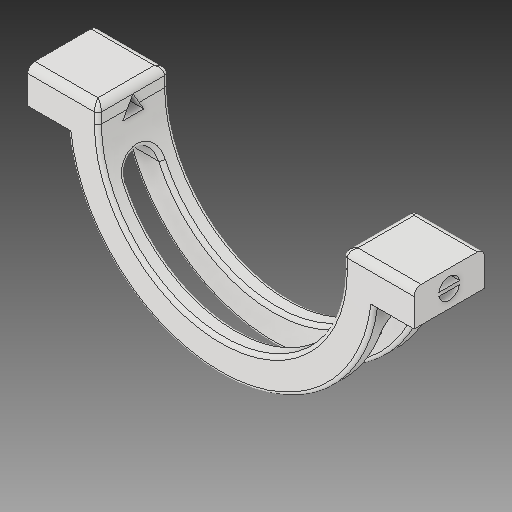
# Autodesk Inventor part: TopCircleArm
Saved by Autodesk Inventor 2017 (Build 210142000, 142)
## iProperties
Created: 2017-02-18
Part Number: TopCircleArm
Material: ABS Plastic
Document SubType Name: Modeling
Designer: aribu
Density: 1.06 g/cm^3
Appearance: Smooth - White
Mass: 19.458 g
Surface Area: 97.5745 cm^2
Volume: 18.3566 cm^3
Author: aribu
Autodesk Inventor part; units mm, degrees
ref_plane "YZ Plane" through (0, 0, 0) normal (1, 0, 0) x (0, 1, 0)
ref_plane "XZ Plane" through (0, 0, 0) normal (0, 1, 0) x (-1, 0, 0)
ref_plane "XY Plane" through (0, 0, 0) normal (0, 0, 1) x (1, 0, 0)
sketch "Sketch1" plane through (0, 0, 0) normal (0, 0, 1) x (1, 0, 0)
  arc A0 (-35, 0) -> (35, 0) centre (0, 0) ccw
  arc A1 (-43.715, -5) -> (43.715, -5) centre (0, 0) ccw
  line L0 (-35, 0) -> (-35, 5)
  line L1 (35, 0) -> (35, 5)
  line L2 (-35, 5) -> (-55, 5)
  line L3 (-55, 5) -> (-55, -5)
  line L4 (-55, -5) -> (-43.715, -5)
  line L5 (35, 5) -> (55, 5)
  line L6 (55, 5) -> (55, -5)
  line L7 (55, -5) -> (43.715, -5)
  dimension "d0" = 70
  dimension "d1" = 88
  dimension "d12" = 20
  dimension "d13" = 20
  dimension "d27" = 10
  dimension "d28" = 10
  constraints: 16 end point, 4 perpendicular, 4 point on circle, 2 centre point, 2 coincident, 2 tangent, 1 horizontal, 1 vertical
  measures "d0" diameter of A0
  measures "d1" diameter of A1
  measures "d12" distance of L0.end L2.end
  measures "d13" distance of L1.end L5.end
  measures "d27" distance of L5.end L6.end
  measures "d28" distance of L2.end L3.end
extrude "Extrusion1" add sketch "Sketch1" along normal blind 20
sketch "Sketch2" plane through (55, -5, 0) normal (1, 0, 0) x (0, 0, -1)
  arc A0 (-5, -10) -> (-15, -10) centre (-10, -10) ccw
  line L0 (0, 10) -> (0, 0)
  line L1 (0, 0) -> (-10, 0)
  line L2 (-15, -10) -> (-15, -42.0097)
  line L3 (-15, -42.0097) -> (-5, -42.0097)
  line L4 (-5, -42.0097) -> (-5, -10)
  line L5 (0, 0) -> (-20, 0) projected
  line L6 (0, 10) -> (0, 0) projected
  dimension "d6" = 10
  dimension "d7" = 10
  dimension "d8" = 10
  dimension "d14" = 0
  dimension "d15" = 0
  dimension "d16" = 10
  constraints: 10 end point, 2 point on circle, 2 tangent, 1 centre point, 1 perpendicular, 1 vertical
  measures "d6" diameter of A0
  measures "d7" distance from line of L0 A0.centre
  measures "d8" distance from line of L1 A0.centre
  measures "d14" distance between parallel lines of L1 L5
  measures "d15" distance between parallel lines of L6 L0
  measures "d16" distance of L2.end L3.end
extrude "Extrusion2" cut sketch "Sketch2" against normal blind 120
fillet "Fillet1" radius 1 16 edges at (33.541, -10, 9.9987) (0, -35, 15) (-33.541, -10, 9.9987) (0, -35, 5) (-42.8486, -10, 9.9954) (0, -44, 15) (42.8486, -10, 9.9954) (0, -44, 5) (0, -44, 20) (0, -44, 0) (35, 2.5, 0) (-35, 2.5, 0) (0, -35, 0) (-35, 2.5, 20) (35, 2.5, 20) (0, -35, 20)
sketch "Sketch3" plane through (55, -5, 0) normal (1, 0, 0) x (0, 0, -1)
  line L0 (-20, 0) -> (-20, 10) projected
  line L1 (0, 10) -> (-20, 10) projected
  line L2 (-12.9139, 4.5) -> (-7.0861, 4.5)
  line L3 (-7.052, 5.5) -> (-12.948, 5.5)
  arc A0 (-12.9139, 4.5) -> (-7.0861, 4.5) centre (-10, 5) ccw
  arc A1 (-7.052, 5.5) -> (-12.948, 5.5) centre (-10, 5) ccw
  point P0 (0, 5)
  dimension "d18" = 10
  dimension "d19" = 5
  dimension "d35" = 1
  dimension "d36" = 0.5
  constraints: 4 end point, 4 point on circle, 2 centre point, 1 horizontal, 1 parallel
  measures "d18" distance from line of L0 A0.centre
  measures "d19" distance from line of A0.centre L1
  measures "d35" distance between parallel lines of L3 L2
  measures "d36" distance from line of L3 A0.centre
extrude "Extrusion3" cut sketch "Sketch3" against normal blind 25
fillet "Fillet2" radius 2 10 edges at (-35.2929, 5, 0.2929) (-35, 5, 10) (-35.2929, 5, 19.7071) (-45.5, 5, 20) (-45.5, 5, 0) (35.2929, 5, 0.2929) (35, 5, 10) (35.2929, 5, 19.7071) (45.5, 5, 20) (45.5, 5, 0)
sketch "Sketch4" plane through (-55, -5, 0) normal (-1, 0, 0) x (0, 0, 1)
  line L0 (19, 8) -> (1, 8) projected
  line L1 (10, 8) -> (7, 2.8038)
  line L2 (7, 2.8038) -> (13, 2.8038)
  line L3 (13, 2.8038) -> (10, 8)
  point P0 (0, 5)
  dimension "d30" = 6
  dimension "d31" = 6
  dimension "d32" = 6
  constraints: 6 end point, 1 horizontal, 1 midpoint
  measures "d30" distance of L2.end L1.start
  measures "d31" distance of L1.start L1.end
  measures "d32" distance of L1.end L2.end
extrude "Extrusion4" cut sketch "Sketch4" against normal blind 25
equation "\"d16\" = d6"
equation "\"d36\" = 0.5 * d35"
body "Solid1"
